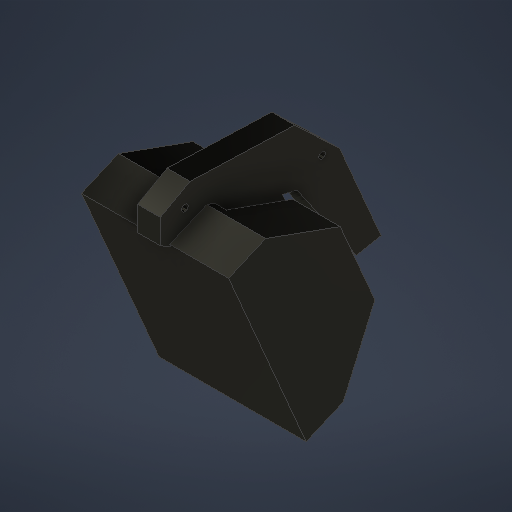
# Autodesk Inventor part: F3 Front Caliper Bracket
Saved by Autodesk Inventor 2026.1 (Build 301233000, 233)
## iProperties
Created: 2026-06-24
Part Number: F3 Front Caliper Bracket
Material: Generic
Document SubType Name: Modeling
Designer: share
Density: 1 g/cm^3
Appearance: Default
Author: share
Autodesk Inventor part; units mm, degrees
ref_plane "YZ Plane" through (0, 0, 0) normal (1, 0, 0) x (0, 1, 0)
ref_plane "XZ Plane" through (0, 0, 0) normal (0, 1, 0) x (-1, 0, 0)
ref_plane "XY Plane" through (0, 0, 0) normal (0, 0, 1) x (1, 0, 0)
sketch "Sketch1" plane through (0, 0, 0) normal (1, 0, 0) x (0, 1, 0)
  line L0 (90, 0) -> (0, 0) construction
  line L1 (0, 0) -> (0, -135) construction
  line L2 (0, -135) -> (90, -135) construction
  line L3 (90, -135) -> (90, 0) construction
  line L4 (80, 0) -> (65, 0)
  line L5 (80, 0) -> (90, -18.1711)
  line L6 (90, -18.1711) -> (87.7664, -82.1322)
  line L7 (87.7664, -82.1322) -> (61.6218, -109.7086)
  line L8 (2.8311, -135) -> (0, -119.8888)
  line L9 (52.695, -83.5675) -> (60.7393, -49.8037)
  line L10 (60.7393, -49.8037) -> (55.0089, -17.3051)
  line L11 (55.0089, -17.3051) -> (65, 0)
  line L12 (55.0089, -17.3051) -> (52.695, -83.5675) construction
  line L13 (52.695, -83.5675) -> (0, -119.8888)
  line L14 (2.8311, -135) -> (61.6218, -109.7086)
  line L15 (87.7664, -82.1322) -> (0, -119.8888) construction
  line L16 (80, 0) -> (61.6218, -109.7086) construction
  line L17 (0, 27) -> (0, -162) projected
  line L18 (-18, 0) -> (108, 0) projected
  circle A0 centre (77.4826, -15.0279) radius 2
  circle A1 centre (63.4392, -98.8597) radius 2
  line L19 (61.6218, -109.7086) -> (23.93, -103.3945) construction
  dimension "d10" = 135
  dimension "d11" = 90
  dimension "d29" = 10
  dimension "d30" = 15
  dimension "d31" = 2
  dimension "d34" = 120
  dimension "d37" = 64
  dimension "d39" = 35
  dimension "d40" = 140
  dimension "d42" = 38
  dimension "d43" = 15
  dimension "d44" = 64
  dimension "d45" = 64
  dimension "d46" = 33
  dimension "d47" = 34.7088
  dimension "d59" = 85
  dimension "d60" = 11
  dimension "d61" = 4
  constraints: 36 end point, 8 point on line, 4 parallel, 2 centre point, 2 collinear, 2 perpendicular, 1 equal radius, 1 horizontal
  measures "d10" distance between parallel lines of L2 L0
  measures "d11" distance between parallel lines of L1 L3
  measures "d29" distance from line of L3 L4.start
  measures "d30" distance of L4.start L4.end
  measures "d31" angle of L3 L6
  measures "d34" angle of L11 L0
  measures "d37" distance of L5.end L6.end
  measures "d39" distance between parallel lines of L12 L6
  measures "d40" angle of L10 L11
  measures "d42" distance of L6.end L7.end
  measures "d43" distance between parallel lines of L14 L15
  measures "d44" distance of L8.start L7.end
  measures "d45" distance of L9.start L8.end
  measures "d46" distance of L9.end L10.end
  measures "d47" distance of L9.start L9.end
  measures "d59" distance of A1.centre A0.centre
  measures "d60" distance from line of L19 A1.centre
  measures "d61" diameter of A0
extrude "Extrusion1" add sketch "Sketch1" along normal blind 14 contours L5 L6 L7 L14 L8 L13 L9 L10 L11 L4
sketch "Sketch2" plane through (0, 0, 0) normal (-1, 0, 0) x (0, 0, 1)
  line L0 (-18.1711, 90) -> (0, 80) projected
  line L1 (-82.1322, 87.7664) -> (-18.1711, 90) projected
  line L2 (-109.7086, 61.6218) -> (-82.1322, 87.7664) projected
  line L3 (-135, 2.8311) -> (-109.7086, 61.6218) projected
  line L4 (-119.8888, 0) -> (-135, 2.8311) projected
  line L5 (-83.5675, 52.695) -> (-119.8888, 0) projected
  line L6 (-49.8037, 60.7393) -> (-83.5675, 52.695) projected
  line L7 (-17.3051, 55.0089) -> (-49.8037, 60.7393) projected
  line L8 (0, 65) -> (-17.3051, 55.0089) projected
  line L9 (0, 80) -> (0, 65) projected
  circle A0 centre (-98.8597, 63.4392) radius 2 projected
  circle A1 centre (-15.0279, 77.4826) radius 2 projected
  line L10 (-135, 2.8311) -> (-109.7086, 61.6218) projected
  line L11 (-18.1711, 90) -> (0, 80) projected
  line L12 (-5.748, 62.8835) -> (-60.8643, 86.5942)
  line L13 (-60.8643, 86.5942) -> (-108.2857, -23.6383)
  line L14 (-108.2857, -23.6383) -> (-53.1695, -47.349)
  line L15 (-53.1695, -47.349) -> (-5.748, 62.8835)
  line L16 (-18.1711, 90) -> (-27.3572, 93.9518)
  point P0 (-74.5203, 54.8505)
  point P1 (-6.436, 61.2841)
  dimension "d70" = 35
  dimension "d72" = 120
  dimension "d76" = 60
  dimension "d78" = 10
  dimension "d79" = 20
  constraints: 10 end point, 3 parallel, 2 perpendicular
  measures "d70" distance between parallel lines of L13 L3
  measures "d72" distance between parallel lines of L12 L14
  measures "d76" distance between parallel lines of L15 L13
  measures "d78" distance of L0.start L16.end
  measures "d79" distance between parallel lines of L16 L12
extrude "Extrusion2" add sketch "Sketch2" along normal blind 40 and the other way blind 50 contours L15 L14 L13 L6 L7 L8 | L8 L7 L6 L13 L12 L15
sketch "Sketch3" plane through (-40, 0, 0) normal (-1, 0, 0) x (0, 0, 1)
  circle A0 centre (-15.0279, 77.4826) radius 2 projected
  line L0 (-83.5675, 52.695) -> (-15.0279, 77.4826)
  line L1 (-5.748, 62.8835) -> (-60.8643, 86.5942) projected
  line L2 (-60.8643, 86.5942) -> (-108.2857, -23.6383) projected
  line L3 (-5.748, 62.8835) -> (-53.1695, -47.349) projected
  line L4 (-29.4587, 7.7672) -> (-84.575, 31.4779) construction
  line L5 (-99.2863, 16.1562) -> (-70.1502, -50.6509)
  line L6 (-108.2857, -23.6383) -> (-53.1695, -47.349) projected
  point P0 (0, 0)
  point P1 (-73.9515, 56.1726)
  point P2 (-28.423, 72.6381)
  point P3 (-75.8445, -37.5944)
  point P4 (-95.1985, 6.7833)
  constraints: 6 end point, 2 midpoint, 2 symmetric about line
extrude "Extrusion3" cut sketch "Sketch3" against normal up to surface (40 mm away) contours L2 L1 L0 | L5 L6 L2
sketch "Sketch4" plane through (50, 0, 0) normal (1, 0, 0) x (0, 0, -1)
  line L0 (5.748, 62.8835) -> (60.8643, 86.5942) projected
  line L1 (60.8643, 86.5942) -> (108.2857, -23.6383) projected
  line L2 (28.423, 72.6381) -> (73.9515, 56.1726) projected
  line L3 (99.2863, 16.1562) -> (70.1502, -50.6509) projected
  line L4 (108.2857, -23.6383) -> (53.1695, -47.349) projected
  point P0 (0, 0)
  point P1 (75.8445, -37.5944)
  point P2 (95.1985, 6.7833)
extrude "Extrusion4" cut sketch "Sketch4" against normal up to surface (36 mm away)
sketch "Sketch5" plane through (14, 0, 0) normal (-1, 0, 0) x (0, 0, 1)
  circle A0 centre (-158.0633, 63.0922) radius 125
  line L0 (-29.4587, 7.7672) -> (-84.575, 31.4779) construction
  line L1 (-84.575, 31.4779) -> (-158.0633, 63.0922)
  point P0 (0, 0)
  dimension "d88" = 80
  dimension "d89" = 250
  constraints: 2 end point, 1 centre point, 1 collinear
  measures "d88" distance of L0.end L1.end
  measures "d89" diameter of A0
extrude "Extrusion5" cut sketch "Sketch5" against normal blind 7
equation "\"d61\" = Mount_Hole_Diameter"
equation "\"Mount_Hole_Diameter\" = 4"
body "Solid1"
